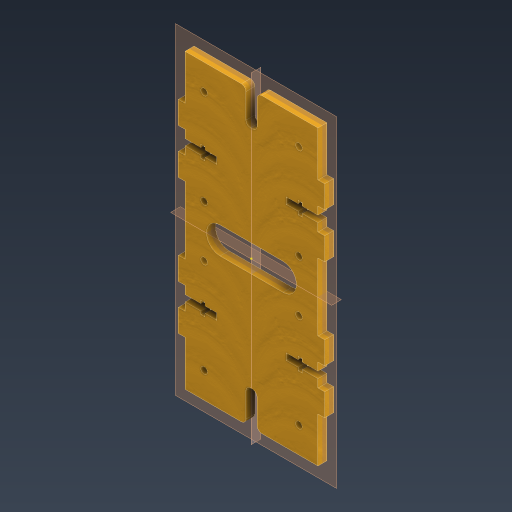
# Autodesk Inventor part: Фанерка ерпления колонок
Saved by Autodesk Inventor 2023.2 (Build 272271030, 271C)
## iProperties
Created: 2024-03-22
Part Number: Фанерка ерпления колонок
Material: Типовые
Document SubType Name: Modeling
Designer: I9232
Density: 1 g/cm^3
Appearance: Сварка — латунь
Author: I9232
Autodesk Inventor part; units mm, degrees
sketch "Эскиз1" plane through (0, 0, 0) normal (0, 0, 1) x (1, 0, 0)
  line L0 (-29.5, -65) -> (29.5, -65)
  line L1 (29.5, -65) -> (29.5, 65)
  line L2 (29.5, 65) -> (-29.5, 65)
  line L3 (-29.5, 65) -> (-29.5, -65)
  line L4 (-29.5, -65) -> (29.5, 65) construction
  line L5 (29.5, -65) -> (-29.5, 65) construction
  point P0 (0, 0)
  dimension "d0" = 59
  dimension "d1" = 130
  constraints: 12 end point, 2 midpoint, 2 parallel, 1 horizontal, 1 perpendicular
  measures "d0" distance of L1.end L2.end
  measures "d1" distance of L0.end L1.end
extrude "Выдавливание1" add sketch "Эскиз1" along normal mid plane 4
sketch "Эскиз3" plane through (-29.5, -65, 2) normal (-1, 0, 0) x (0, 0, 1)
  line L0 (-4, 0) -> (-4, 130) projected
  line L1 (0, 0) -> (0, 130) projected
  line L2 (-4, 100) -> (0, 100)
  line L3 (0, 100) -> (0, 110)
  line L4 (0, 110) -> (-4, 110)
  line L5 (-4, 110) -> (-4, 100)
  line L6 (-4, 130) -> (0, 130) projected
  line L7 (-4, 90) -> (0, 90)
  line L8 (0, 90) -> (0, 80)
  line L9 (0, 80) -> (-4, 80)
  line L10 (-4, 80) -> (-4, 90)
  line L11 (-4, 65) -> (0, 65) construction
  line L12 (-4, 30) -> (0, 30)
  line L13 (0, 30) -> (0, 20)
  line L14 (0, 20) -> (-4, 20)
  line L15 (-4, 20) -> (-4, 30)
  line L16 (-4, 40) -> (0, 40)
  line L17 (0, 40) -> (0, 50)
  line L18 (0, 50) -> (-4, 50)
  line L19 (-4, 50) -> (-4, 40)
  point P0 (-2, 65)
  point P1 (0, 30)
  point P2 (0, 40)
  point P3 (0, 90)
  point P4 (0, 100)
  dimension "d18" = 10
  dimension "d19" = 10
  dimension "d20" = 20
  dimension "d21" = 10
  constraints: 34 end point, 8 symmetric about line, 4 parallel, 4 point on line, 2 horizontal, 2 midpoint, 2 perpendicular
  measures "d18" distance between parallel lines of L7 L2
  measures "d19" distance of L8.end L7.end
  measures "d20" distance between parallel lines of L6 L4
  measures "d21" distance of L2.end L3.end
extrude "Выдавливание3" add sketch "Эскиз3" along normal blind 3 contours L0 L12 L1 L14 | L0 L18 L1 L16 | L0 L7 L1 L9 | L0 L4 L1 L2
mirror "Зеркальное отражение2" about plane through (0, 0, 0) normal (1, 0, 0) of "Выдавливание3"
sketch "Эскиз4" plane through (0, 0, 2) normal (0, 0, 1) x (1, 0, 0)
  line L0 (-15.4, 31.45) -> (-15.4, 28.55)
  line L1 (-29.5, 28.55) -> (-29.5, 31.45)
  line L2 (-22.5, 32.8) -> (-20.7, 32.8)
  line L3 (-22.5, 27.2) -> (-20.7, 27.2)
  line L4 (-29.5, 30) -> (-15.4, 30)
  line L5 (-20.7, 27.2) -> (-20.7, 28.55)
  line L6 (-22.5, 31.45) -> (-22.5, 32.8)
  line L7 (-20.7, 32.8) -> (-20.7, 31.45)
  line L8 (-22.5, 28.55) -> (-22.5, 27.2)
  line L9 (-29.5, 31.45) -> (-22.5, 31.45)
  line L10 (-20.7, 31.45) -> (-15.4, 31.45)
  line L11 (-15.4, 28.55) -> (-20.7, 28.55)
  line L12 (-22.5, 28.55) -> (-29.5, 28.55)
  line L13 (-29.5, 35) -> (-29.5, 25) projected
  line L14 (0, 3.054) -> (0, -3.054) construction
  line L15 (-15.3649, 0) -> (15.3649, 0)
  line L16 (-15.4, -31.45) -> (-15.4, -28.55)
  line L17 (-29.5, -28.55) -> (-29.5, -31.45)
  line L18 (-22.5, -32.8) -> (-20.7, -32.8)
  line L19 (-22.5, -27.2) -> (-20.7, -27.2)
  line L20 (-29.5, -30) -> (-15.4, -30)
  line L21 (-20.7, -27.2) -> (-20.7, -28.55)
  line L22 (-22.5, -31.45) -> (-22.5, -32.8)
  line L23 (-20.7, -32.8) -> (-20.7, -31.45)
  line L24 (-22.5, -28.55) -> (-22.5, -27.2)
  line L25 (-29.5, -31.45) -> (-22.5, -31.45)
  line L26 (-20.7, -31.45) -> (-15.4, -31.45)
  line L27 (-15.4, -28.55) -> (-20.7, -28.55)
  line L28 (-22.5, -28.55) -> (-29.5, -28.55)
  line L29 (-29.5, -35) -> (-29.5, -25)
  line L30 (0, -3.054) -> (0, 3.054) construction
  line L31 (15.4, 31.45) -> (15.4, 28.55)
  line L32 (29.5, 28.55) -> (29.5, 31.45)
  line L33 (22.5, 32.8) -> (20.7, 32.8)
  line L34 (22.5, 27.2) -> (20.7, 27.2)
  line L35 (29.5, 30) -> (15.4, 30)
  line L36 (20.7, 27.2) -> (20.7, 28.55)
  line L37 (22.5, 31.45) -> (22.5, 32.8)
  line L38 (20.7, 32.8) -> (20.7, 31.45)
  line L39 (22.5, 28.55) -> (22.5, 27.2)
  line L40 (29.5, 31.45) -> (22.5, 31.45)
  line L41 (20.7, 31.45) -> (15.4, 31.45)
  line L42 (15.4, 28.55) -> (20.7, 28.55)
  line L43 (22.5, 28.55) -> (29.5, 28.55)
  line L44 (29.5, 35) -> (29.5, 25)
  line L45 (20.7, -27.2) -> (20.7, -28.55)
  line L46 (22.5, -27.2) -> (20.7, -27.2)
  line L47 (22.5, -28.55) -> (22.5, -27.2)
  line L48 (20.7, -31.45) -> (15.4, -31.45)
  line L49 (20.7, -32.8) -> (20.7, -31.45)
  line L50 (22.5, -32.8) -> (20.7, -32.8)
  line L51 (22.5, -31.45) -> (22.5, -32.8)
  line L52 (29.5, -30) -> (15.4, -30)
  line L53 (22.5, -28.55) -> (29.5, -28.55)
  line L54 (29.5, -28.55) -> (29.5, -31.45)
  line L55 (29.5, -31.45) -> (22.5, -31.45)
  line L56 (15.4, -31.45) -> (15.4, -28.55)
  line L57 (15.4, -28.55) -> (20.7, -28.55)
  point P0 (0, 0)
  point P1 (0, 0)
  point P2 (29.5, -25)
  dimension "d26" = 2.9
  dimension "d31" = 1.8
  dimension "d32" = 1.35
  dimension "d33" = 7
  dimension "d34" = 5.3
  dimension "d35" = 2.9
  constraints: 114 end point, 49 symmetric about line, 8 parallel, 5 midpoint, 4 equal length, 4 horizontal, 4 perpendicular, 2 collinear, 1 coincident, 1 vertical
  measures "d26" distance of L0.end L0.start
  measures "d31" distance of L2.start L2.end
  measures "d32" distance of L2.end L7.end
  measures "d33" distance of L1.end L6.start
  measures "d34" distance between parallel lines of L0 L7
  measures "d35" distance of L1.start L1.end
extrude "Выдавливание4" cut sketch "Эскиз4" against normal up to surface (4 mm away)
sketch "Эскиз5" plane through (0, 0, 2) normal (0, 0, 1) x (1, 0, 0)
  line L0 (29.5, 65) -> (-29.5, 65) construction
  line L1 (2.5, 65) -> (-2.5, 65)
  line L2 (-2.5, 65) -> (-2.5, 50)
  line L3 (-2.5, 50) -> (2.5, 50)
  line L4 (2.5, 50) -> (2.5, 65)
  line L5 (-2.9793, 0) -> (2.9793, 0) construction
  line L6 (29.5, -65) -> (-29.5, -65) construction
  line L7 (-2.5, -65) -> (-2.5, -50)
  line L8 (-2.5, -50) -> (2.5, -50)
  line L9 (2.5, -50) -> (2.5, -65)
  line L10 (-2.5, -65) -> (2.5, -65)
  line L11 (-29.5, -65) -> (29.5, -65) projected
  point P0 (0, 0)
  point P1 (0, 65)
  point P2 (0, 0)
  dimension "d38" = 5
  dimension "d39" = 15
  constraints: 20 end point, 6 symmetric about line, 3 midpoint, 2 horizontal, 2 parallel, 2 point on line, 1 coincident, 1 collinear, 1 perpendicular
  measures "d38" distance of L2.end L3.end
  measures "d39" distance of L3.end L1.start
extrude "Выдавливание5" cut sketch "Эскиз5" against normal up to surface (4 mm away)
fillet "Сопряжение1" radius 2 8 edges at (2.5, 50, 0) (-2.5, 50, 0) (-2.5, -50, 0) (2.5, -50, 0) (2.5, 65, 0) (-2.5, 65, 0) (2.5, -65, 0) (-2.5, -65, 0)
sketch "Эскиз8" plane through (0, 0, 2) normal (0, 0, 1) x (1, 0, 0)
  circle A0 centre (-21.05, 11.45) radius 1.5
  circle A1 centre (21.05, 11.45) radius 1.5
  circle A2 centre (-21.05, 53.55) radius 1.5
  circle A3 centre (21.05, 53.55) radius 1.5
  circle A4 centre (21.05, -11.45) radius 1.5
  circle A5 centre (-21.05, -11.45) radius 1.5
  circle A6 centre (-21.05, -53.55) radius 1.5
  circle A7 centre (21.05, -53.55) radius 1.5
  point P0 (0, 0)
  constraints: 8 centre point
extrude "Выдавливание8" cut sketch "Эскиз8" against normal up to surface (4 mm away)
sketch "Эскиз9" plane through (0, 0, 2) normal (0, 0, 1) x (1, 0, 0)
  point P0 (0, 0)
sketch "Эскиз10" plane through (0, 0, 2) normal (0, 0, 1) x (1, 0, 0)
  line L0 (-14, 0) -> (14, 0) construction
  line L1 (-14, -6) -> (14, -6)
  line L2 (14, 6) -> (-14, 6)
  arc A0 (-14, 6) -> (-14, -6) centre (-14, 0) ccw
  arc A1 (14, -6) -> (14, 6) centre (14, 0) ccw
  point P0 (0, 0)
  point P1 (-20, 0)
  point P2 (20, 0)
  dimension "d49" = 12
  dimension "d50" = 40
  constraints: 8 end point, 6 point on circle, 4 tangent, 2 centre point, 1 horizontal, 1 midpoint, 1 parallel
  measures "d49" distance between parallel lines of L1 L2
  measures "d50" distance of point (-20, 0) point (20, 0)
extrude "Выдавливание9" cut sketch "Эскиз10" against normal up to next
